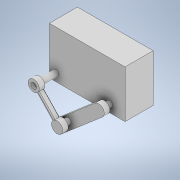
# Autodesk Inventor part: Деталь3
Saved by Autodesk Inventor 2020.1 (Build 241239000, 239)
## iProperties
Created: 2021-11-17
Part Number: Деталь3
Material: Типовые
Document SubType Name: Modeling
Designer: Ni3na
Density: 1 g/cm^3
Appearance: По умолчанию
Author: Ni3na
Autodesk Inventor part; units mm, degrees
ref_plane "YZ Plane" through (0, 0, 0) normal (1, 0, 0) x (0, 1, 0)
ref_plane "XZ Plane" through (0, 0, 0) normal (0, 1, 0) x (-1, 0, 0)
ref_plane "XY Plane" through (0, 0, 0) normal (0, 0, 1) x (1, 0, 0)
sketch "Эскиз1" plane through (0, 0, 0) normal (0, 0, 1) x (1, 0, 0)
  line L0 (10.0582, -8.8009) -> (-16.8718, -8.8009)
  line L1 (-16.8718, -8.8009) -> (-16.8718, 8.0709)
  line L2 (-16.8718, 8.0709) -> (10.0582, 8.0709)
  line L3 (10.0582, 8.0709) -> (10.0582, -8.8009)
  point P0 (0, 0)
  constraints: 8 end point, 2 parallel, 1 horizontal, 1 perpendicular
extrude "Выдавливание1" add sketch "Эскиз1" along normal blind 10
sketch "Эскиз2" plane through (0, 0, 10) normal (0, 0, 1) x (1, 0, 0)
  circle A0 centre (4.6641, -5.9619) radius 1
  circle A1 centre (-14.4383, -5.9619) radius 1
  point P0 (0, 0)
  dimension "d2" = 2
  dimension "d3" = 2
  constraints: 2 centre point
  measures "d2" diameter of A0
  measures "d3" diameter of A1
extrude "Выдавливание2" add sketch "Эскиз2" along normal blind 2
sketch "Эскиз3" plane through (4.6641, -5.9619, 12) normal (0, 0, 1) x (1, 0, 0)
  circle A0 centre (0, 0) radius 1 projected
  circle A1 centre (0, 0) radius 2
  circle A2 centre (-14.7836, -12.664) radius 2
  line L0 (-1.2061, 1.5954) -> (-15.8126, -10.949)
  line L1 (-13.5836, -14.264) -> (1.0265, -1.7165)
  point P0 (-4.6641, 5.9619)
  dimension "d6" = 4
  dimension "d7" = 4
  constraints: 4 end point, 4 point on circle, 2 centre point, 1 coincident, 1 parallel
  measures "d6" diameter of A1
  measures "d7" diameter of A2
extrude "Выдавливание3" add sketch "Эскиз3" along normal blind 2 contours A0 | A1 | A1 L1 A2 L0
sketch "Эскиз4" plane through (-14.4383, -5.9619, 12) normal (0, 0, 1) x (1, 0, 0)
  circle A0 centre (0, 0) radius 1
  point P0 (14.4383, 5.9619)
  constraints: 1 centre point
extrude "Выдавливание4" add sketch "Эскиз4" along normal blind 4
sketch "Эскиз5" plane through (4.6641, -5.9619, 14) normal (0, 0, 1) x (1, 0, 0)
  circle A0 centre (-10.7969, -8.6603) radius 1
  point P0 (-4.6641, 5.9619)
  dimension "d12" = 2
  constraints: 1 centre point
  measures "d12" diameter of A0
extrude "Выдавливание5" add sketch "Эскиз5" along normal blind 2
sketch "Эскиз6" plane through (4.6641, -5.9619, 14) normal (0, 0, 1) x (1, 0, 0)
  circle A0 centre (-15.0265, -12.7992) radius 1
  point P0 (-4.6641, 5.9619)
  dimension "d15" = 2
  constraints: 1 centre point
  measures "d15" diameter of A0
extrude "Выдавливание6" cut sketch "Эскиз6" against normal blind 10
sketch "Эскиз7" plane through (-14.4383, -5.9619, 16) normal (0, 0, 1) x (1, 0, 0)
  circle A0 centre (0, 0) radius 2
  circle A1 centre (8.3055, -8.6603) radius 1 projected
  circle A2 centre (8.3055, -8.6603) radius 2
  line L0 (7.3055, -6.9282) -> (1.7093, -1.0384)
  line L1 (6.6268, -7.5731) -> (1.0492, -1.7027)
  point P0 (14.4383, 5.9619)
  dimension "d18" = 4
  dimension "d19" = 4
  constraints: 4 end point, 4 point on circle, 2 centre point, 1 coincident, 1 parallel
  measures "d18" diameter of A0
  measures "d19" diameter of A2
extrude "Выдавливание7" add sketch "Эскиз7" along normal blind 2 contours A0 | A0 L0 A2 L1 | A2 | A1
sketch "Эскиз8" plane through (-14.4383, -5.9619, 18) normal (0, 0, 1) x (1, 0, 0)
  circle A0 centre (0, 0) radius 1
  point P0 (14.4383, 5.9619)
  constraints: 1 centre point
extrude "Выдавливание8" cut sketch "Эскиз8" against normal blind 1
chamfer "Фаска1" distance 0.3 angle 45 4 edges at (-9.9309, -9.9452, 18) (-9.9309, -9.9452, 16) (-10.6004, -10.5998, 16) (-10.6004, -10.5998, 18)
